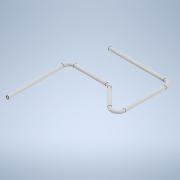
# Autodesk Inventor part: Tubo
Saved by Autodesk Inventor 2021 (Build 250183000, 183)
## iProperties
Created: 2021-05-06
Part Number: Tubo
Material: Genérico
Document SubType Name: Modeling
Designer: rubia
Density: 1 g/cm^3
Appearance: Padrão
Author: rubia
Autodesk Inventor part; units mm, degrees
ref_plane "YZ Plane" through (0, 0, 0) normal (1, 0, 0) x (0, 1, 0)
ref_plane "XZ Plane" through (0, 0, 0) normal (0, 1, 0) x (-1, 0, 0)
ref_plane "Plano de trabalho1" through (0, -0.1328, 0) normal (1, 0, 0) x (0, 1, 0)
sketch "Esboço1" plane through (0, -0.1328, 0) normal (1, 0, 0) x (0, 1, 0)
  circle A0 centre (0.1328, 0) radius 0.5
  circle A1 centre (0.1328, 0) radius 0.75
  dimension "d9" = 1
  dimension "d10" = 1.5
  constraints: 2 centre point, 2 coincident
  measures "d9" diameter of A0
  measures "d10" diameter of A1
sketch3d "Esboço 3D1"
  line L0 (0, -0.1328, 0) -> (27, -0.1328, 0)
  arc A0 (27, -0.1328, 0) -> (30, -0.1328, 3) centre (27, -0.1328, 3) ccw
  line L1 (30, -0.1328, 3) -> (30, -0.1328, 22.8231)
  arc A1 (30, -0.1328, 22.8231) -> (24.8924, -0.1328, 24.9581) centre (27, -0.1328, 22.8231) ccw
  line L2 (24.8924, -0.1328, 24.9581) -> (16.643, -0.1328, 16.8146)
  arc A2 (16.643, -0.1328, 16.8146) -> (14.5354, -0.1328, 15.9496) centre (14.5354, -0.1328, 18.9496) ccw
  line L3 (14.5354, -0.1328, 15.9496) -> (-1.2333, -0.1328, 15.9496)
  arc A3 (-1.2333, -0.1328, 15.9496) -> (-4.2333, -0.1328, 18.9496) centre (-1.2333, -0.1328, 18.9496) ccw
  line L4 (-4.2333, -0.1328, 18.9496) -> (-4.2333, -0.1328, 45.9496)
  dimension "d0" = 30
  dimension "d1" = 30
  dimension "d2" = 20
  dimension "d3" = 20
  dimension "d4" = 30
  dimension "d5" = 3
  dimension "d6" = 3
  dimension "d7" = 3
  dimension "d8" = 3
sweep "Varredura1" add profiles "Esboço1" path "Esboço 3D1"
equation "\"d6\" = d5"
equation "\"d7\" = d5"
equation "\"d8\" = d5"
